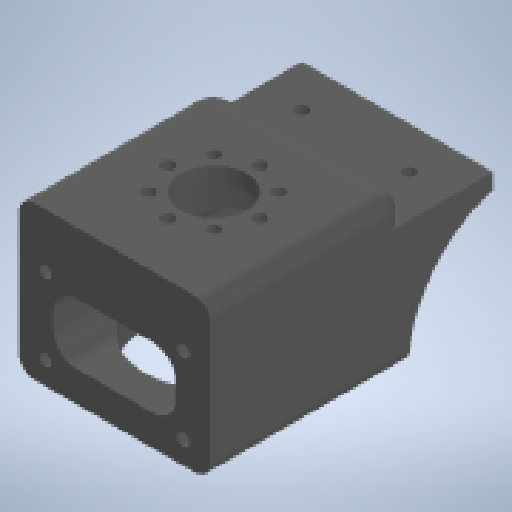
# Autodesk Inventor part: hipjoint_middle
Saved by Autodesk Inventor 2024.1 (Build 281209000, 209)
## iProperties
Created: 2024-02-13
Part Number: hipjoint_middle
Material: 一般
Document SubType Name: モデリング
Designer: hibik
Density: 1 g/cm^3
Appearance: 既定
Author: hibik
Autodesk Inventor part; units mm, degrees
ref_plane "YZ Plane" through (0, 0, 0) normal (1, 0, 0) x (0, 1, 0)
ref_plane "XZ Plane" through (0, 0, 0) normal (0, 1, 0) x (-1, 0, 0)
ref_plane "XY Plane" through (0, 0, 0) normal (0, 0, 1) x (1, 0, 0)
sketch "スケッチ1" plane through (0, 0, 0) normal (0, 0, 1) x (1, 0, 0)
  line L0 (-12.5, 20) -> (12.5, 20)
  circle A0 centre (-9, 13) radius 0.8
  circle A1 centre (9, 13) radius 0.8
  line L1 (-12.5, 20) -> (-12.5, 0)
  line L2 (-12.5, 0) -> (12.5, 0)
  line L3 (12.5, 0) -> (12.5, 20)
  line L4 (-17.5, 0) -> (17.5, 0) projected
  circle A2 centre (-9, 3) radius 0.8
  circle A3 centre (9, 3) radius 0.8
  point P0 (0, 0)
  point P1 (0, 20)
  point P2 (0, 0)
  dimension "d5" = 1.6
  dimension "d6" = 1.6
  dimension "d9" = 7
  dimension "d10" = 7
  dimension "d53" = 20
  dimension "d54" = 25
  dimension "d55" = 9
  dimension "d56" = 9
  dimension "d57" = 3
  constraints: 8 end point, 4 centre point, 4 vertical alignment, 2 equal radius, 2 midpoint, 1 collinear, 1 horizontal, 1 horizontal alignment, 1 perpendicular, 1 vertical
  measures "d5" diameter of A0
  measures "d6" diameter of A1
  measures "d9" distance from line of L0 A0.centre
  measures "d10" distance from line of L0 A1.centre
  measures "d53" distance of L0.start L1.end
  measures "d54" distance of L0.start L0.end
  measures "d55" horizontal distance of point (0, 20) A0.centre
  measures "d56" horizontal distance of point (0, 20) A1.centre
  measures "d57" distance from line of L2 A2.centre
extrude "押し出し1" add sketch "スケッチ1" along normal blind 26 contours L0 L3 L2 L1 | A0 | A1 | A2 | A3
sketch "スケッチ8" plane through (-12.5, 20, 0) normal (0, 1, 0) x (1, 0, 0)
  circle A0 centre (12.5, -13) radius 4.25
  circle A1 centre (12.5, -13) radius 6 construction
  circle A2 centre (12.5, -13) radius 9
  line L0 (25, 0) -> (25, -26) projected
  line L1 (25, 0) -> (0, 0) projected
  circle A3 centre (12.5, -7) radius 0.8
  circle A4 centre (8.2574, -8.7574) radius 0.8
  circle A5 centre (6.5, -13) radius 0.8
  circle A6 centre (8.2574, -17.2426) radius 0.8
  circle A7 centre (12.5, -19) radius 0.8
  circle A8 centre (16.7426, -17.2426) radius 0.8
  circle A9 centre (18.5, -13) radius 0.8
  circle A10 centre (16.7426, -8.7574) radius 0.8
  point P0 (12.5, 0)
  point P1 (25, -13)
  point P2 (12.5, 0)
  point P3 (12.5, 0)
  dimension "d59" = 12
  dimension "d58" = 8.5
  dimension "d60" = 18
  dimension "d61" = 1.6
  dimension "d64" = 360
  constraints: 10 centre point, 3 midpoint, 3 vertical alignment, 2 coincident, 1 horizontal alignment, 19 other
  measures "d58" diameter of A0
  measures "d60" diameter of A2
  measures "d61" diameter of A3
extrude "押し出し8" cut sketch "スケッチ8" against normal through all contours A0 | A2 | A3 | A4 | A5 | A6 | A7 | A8 | A9 | A10
extrude "押し出し9" add sketch "スケッチ8" against normal blind 2
sketch "スケッチ9" plane through (0, 0, 26) normal (0, 0, 1) x (1, 0, 0)
  line L0 (-9, 13) -> (9, 13) construction
  line L1 (9, 13) -> (9, 3) construction
  line L2 (9, 3) -> (-9, 3) construction
  line L3 (-9, 3) -> (-9, 13) construction
  line L4 (-8, 12) -> (8, 12)
  line L5 (8, 12) -> (8, 4)
  line L6 (8, 4) -> (-8, 4)
  line L7 (-8, 4) -> (-8, 12)
  line L8 (12.5, 20) -> (-12.5, 20) projected
  line L9 (-12.5, 0) -> (12.5, 0) projected
  point P0 (0, 0)
  point P1 (-8, 8)
  point P2 (-9, 8)
  point P3 (0, 12)
  point P4 (0, 13)
  point P5 (0, 20)
  dimension "d70" = 1
  dimension "d71" = 1
  dimension "d80" = 7
  dimension "d81" = 3
  dimension "d82" = 18
  constraints: 16 end point, 5 midpoint, 4 parallel, 2 horizontal, 2 perpendicular, 2 vertical alignment, 1 horizontal alignment
  measures "d70" distance between parallel lines of L0 L4
  measures "d71" distance between parallel lines of L3 L7
  measures "d80" distance between parallel lines of L8 L0
  measures "d81" distance between parallel lines of L9 L2
  measures "d82" distance of L0.start L0.end
extrude "押し出し10" cut sketch "スケッチ9" against normal through all
fillet "フィレット2" radius 3 8 edges at (-8, 12, 21.5616) (8, 12, 21.5616) (8, 4, 21.5616) (-8, 4, 21.5616) (-8, 4, 4.4384) (-8, 12, 4.4384) (8, 12, 4.4384) (8, 4, 4.4384)
fillet "フィレット3" radius 2 4 edges at (12.5, 20, 13) (-12.5, 20, 13) (12.5, 0, 13) (-12.5, 0, 13)
extrude "押し出し11" cut sketch "スケッチ1" along normal blind 8 contours A0 | A1 | A2 | A3
ref_plane "作業平面4" through (0, 0, 13) normal (0, 0, -1) x (-1, 0, 0)
mirror "ミラー1" about plane through (0, 0, 13) normal (0, 0, -1) of "押し出し11"
sketch "スケッチ10" plane through (0, 0, 0) normal (0, 0, -1) x (-1, 0, 0)
  circle A0 centre (-9, 13) radius 0.8 projected
  circle A1 centre (9, 3) radius 0.8 projected
  circle A2 centre (9, 13) radius 0.8 projected
  circle A3 centre (-9, 3) radius 0.8 projected
  line L0 (-8, 7) -> (-8, 9) projected
  arc A4 (-5, 12) -> (-8, 9) centre (-5, 9) ccw projected
  line L1 (-5, 12) -> (5, 12) projected
  arc A5 (8, 9) -> (5, 12) centre (5, 9) ccw projected
  line L2 (8, 9) -> (8, 7) projected
  arc A6 (5, 4) -> (8, 7) centre (5, 7) ccw projected
  line L3 (5, 4) -> (-5, 4) projected
  arc A7 (-8, 7) -> (-5, 4) centre (-5, 7) ccw projected
  arc A8 (10.5, 0) -> (12.5, 2) centre (10.5, 2) ccw projected
  line L4 (12.5, 18) -> (12.5, 2) projected
  arc A9 (12.5, 18) -> (10.5, 20) centre (10.5, 18) ccw projected
  line L5 (-10.5, 20) -> (10.5, 20) projected
  arc A10 (-10.5, 20) -> (-12.5, 18) centre (-10.5, 18) ccw projected
  line L6 (-12.5, 2) -> (-12.5, 18) projected
  arc A11 (-12.5, 2) -> (-10.5, 0) centre (-10.5, 2) ccw projected
  line L7 (10.5, 0) -> (-10.5, 0) projected
  line L8 (-12.5, 16.5) -> (12.5, 16.5)
  point P0 (0, 0)
  dimension "d83" = 3.5
  constraints: 2 end point, 2 point on line, 1 horizontal
  measures "d83" distance between parallel lines of L5 L8
extrude "押し出し12" add sketch "スケッチ10" along normal blind 11 contours A0 | A1 | A2 | A3 | L7 A11 L6 L8 L4 A8
sketch "スケッチ11" plane through (-12.5, 2, 26) normal (-1, 0, 0) x (0, 0, 1)
  line L0 (-37, 0) -> (-37, 14.5) projected
  arc A0 (-26, -2) -> (-37, 12.5) centre (-41.0568, -2) ccw
  line L1 (-37, 12.5) -> (-30.7188, 12.5)
  line L2 (-26, -2) -> (-26, 4.4696)
  line L3 (-26, 14.5) -> (-37, 14.5) projected
  line L4 (-37, 0) -> (-37, -2) projected
  line L5 (0, -2) -> (-37, -2) projected
  dimension "d86" = 2
  constraints: 4 end point, 2 parallel, 2 point on circle, 1 centre point, 1 point on line, 1 tangent
  measures "d86" distance between parallel lines of L3 L1
extrude "押し出し13" cut sketch "スケッチ11" against normal through all
sketch "スケッチ12" plane through (-12.5, 16.5, 0) normal (0, 1, 0) x (1, 0, 0)
  circle A0 centre (19.5, 5.5) radius 0.8
  circle A1 centre (5.5, 5.5) radius 0.8
  circle A2 centre (12.5, -13) radius 4.25 projected
  line L0 (25, 0) -> (25, 11) projected
  point P0 (12.5, 0)
  point P1 (25, 5.5)
  dimension "d89" = 1.6
  dimension "d90" = 7
  dimension "d91" = 7
  constraints: 2 centre point, 2 horizontal alignment, 1 equal radius, 1 midpoint
  measures "d89" diameter of A0
  measures "d90" horizontal distance of A2.centre A0.centre
  measures "d91" horizontal distance of A2.centre A1.centre
extrude "押し出し14" cut sketch "スケッチ12" against normal through all contours A0 | A1
fillet "フィレット4" radius 3 5 edges at (-12.5, 17.25, 0) (-11.9142, 19.4142, 0) (0, 20, 0) (11.9142, 19.4142, 0) (12.5, 17.25, 0)
equation "\"d9\" = d10"
equation "\"d56\" = d55"
equation "\"d71\" = d70"
equation "\"d91\" = d90"
equation "\"BendRadius\" = Thickness"
equation "\"BendReliefWidth\" = Thickness"
equation "\"BendReliefDepth\" = 0.5 * Thickness"
equation "\"CornerReliefSize\" = 4 * Thickness"
equation "\"MinimumRemnant\" = 2 * Thickness"
equation "\"TransitionRadius\" = BendRadius"
equation "\"JacobiRadiusSize\" = BendRadius"
equation "\"GapSize\" = Thickness"
equation "\"Thickness\" = 3.048"
